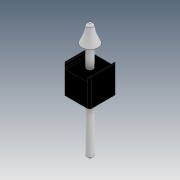
# Autodesk Inventor part: pins
Saved by Autodesk Inventor 2020 (Build 240168000, 168)
## iProperties
Created: 2020-09-27
Part Number: pins
Material: Generic
Document SubType Name: Modeling
Designer: DELL
Density: 1 g/cm^3
Appearance: Default
Author: DELL
Autodesk Inventor part; units mm, degrees
ref_plane "YZ Plane" through (0, 0, 0) normal (1, 0, 0) x (0, 1, 0)
ref_plane "XZ Plane" through (0, 0, 0) normal (0, 1, 0) x (-1, 0, 0)
sketch "Sketch5" plane through (0, 0, 0) normal (0, 1, 0) x (-1, 0, 0)
  line L0 (-1.225, -1.1) -> (1.225, -1.1)
  line L1 (1.225, -1.1) -> (1.225, 1.1)
  line L2 (1.225, 1.1) -> (-1.225, 1.1)
  line L3 (-1.225, 1.1) -> (-1.225, -1.1)
  line L4 (-1.225, -1.1) -> (1.225, 1.1) construction
  line L5 (1.225, -1.1) -> (-1.225, 1.1) construction
  line L6 (1.225, 1.1) -> (1.075, 1.27)
  line L7 (1.075, 1.27) -> (-1.075, 1.27)
  line L8 (-1.075, 1.27) -> (-1.225, 1.1)
  line L9 (0, 1.1) -> (0, -1.1) construction
  line L10 (1.225, 0) -> (-1.225, 0) construction
  line L11 (1.225, -1.1) -> (1.075, -1.27)
  line L12 (1.075, -1.27) -> (-1.075, -1.27)
  line L13 (-1.075, -1.27) -> (-1.225, -1.1)
  point P0 (0, 0)
  dimension "d33" = 2.2
  dimension "d34" = 2.45
  dimension "d36" = 0.15
  dimension "d37" = 2.54
  constraints: 28 end point, 6 midpoint, 2 horizontal, 2 parallel, 2 symmetric about line, 1 perpendicular, 1 other
  measures "d33" distance of L0.end L1.end
  measures "d34" distance between parallel lines of L3 L1
  measures "d36" horizontal distance of L1.end L6.end
  measures "d37" distance between parallel lines of L12 L7
extrude "Extrusion4" add sketch "Sketch5" along normal blind 2.54
sketch "Sketch6" plane through (-1.075, 0, 1.27) normal (0, 0, 1) x (1, 0, 0)
  line L0 (0, 2.54) -> (2.15, 2.54) projected
  line L1 (2.15, 2.14) -> (0, 2.14)
  line L2 (0, 2.14) -> (0, 2.54)
  line L3 (0, 2.54) -> (2.15, 2.54)
  line L4 (2.15, 2.54) -> (2.15, 2.14)
  line L5 (2.15, 2.14) -> (0, 2.54) construction
  line L6 (0, 2.14) -> (2.15, 2.54) construction
  line L7 (1.075, 0) -> (1.075, 2.54) construction
  point P0 (1.075, 2.34)
  dimension "d40" = 2.15
  dimension "d41" = 0.4
  constraints: 14 end point, 3 midpoint, 2 parallel, 2 perpendicular, 1 horizontal, 1 point on line, 1 other
  measures "d40" distance of L1.start L1.end
  measures "d41" distance of L3.end L1.start
extrude "Extrusion5" cut sketch "Sketch6" against normal through all
chamfer "Chamfer3" distance 0.1 angle 45 2 edges at (-1.075, 2.14, 0) (1.075, 2.14, 0)
chamfer "Chamfer4" distance 0.03 angle 45 2 edges at (1.075, 2.54, 0) (-1.075, 2.54, 0)
sketch "Sketch7" plane through (-0.975, 2.14, 1.27) normal (0, 1, 0) x (1, 0, 0)
  circle A0 centre (0.975, 1.27) radius 0.3
  dimension "d50" = 0.6
  constraints: 1 centre point, 1 coincident
  measures "d50" diameter of A0
extrude "Extrusion6" add sketch "Sketch7" along normal blind 3.6 and the other way blind 7.2
chamfer "Chamfer5" distance 0.2 angle 45 2 edges at (-0.3, 5.74, 0) (-0.3, -5.06, 0)
ref_plane "Work Plane1" through (0, 2.14, 0) normal (0, 0, -1) x (0, 1, 0)
sketch "Sketch8" plane through (0, 2.14, 0) normal (0, 0, -1) x (0, 1, 0)
  line L0 (0, -0.3) -> (3.4, -0.3) projected
  line L1 (1.975, -0.75) -> (1.975, 0)
  line L2 (3.4, 0) -> (3.4, -0.3)
  line L3 (0, 0.3) -> (0, -0.3) projected
  line L4 (3.4, -0.3) -> (3.4, 0.3) projected
  line L5 (3.6, 0.1) -> (3.6, -0.1) construction
  line L6 (3.6, 0) -> (0, 0) construction
  line L7 (-9.36, 0) -> (5.76, 0) construction
  line L8 (0.4, -1.225) -> (0.4, -1.105) construction
  line L9 (3.4, -0.3) -> (3.4, 0.3) projected
  line L10 (3.4, 0) -> (1.975, 0)
  line L11 (3.4, -0.3) -> (2.9466, -0.3) construction
  line L12 (2.9466, -0.3) -> (2.3806, -0.5247) construction
  line L13 (2.3806, -0.5247) -> (1.975, -0.75) construction
  spline S0 degree 3 poles (3.4, -0.3) (2.9466, -0.3) (2.3806, -0.5247) (1.975, -0.75) knots 1 1 1 1 2 2 2 2
  point P0 (-2.14, 0)
  point P1 (1.975, -0.3)
  dimension "d59" = 1.575
  dimension "d61" = 0.75
  constraints: 8 end point, 3 midpoint, 2 point on line, 1 collinear, 1 horizontal, 1 parallel, 1 perpendicular, 3 other
  measures "d59" distance between parallel lines of L1 L8
  measures "d61" distance of L1.start L1.end
revolve "Revolution1" add sketch "Sketch8" angle 360 about axis through (0, 2.14, 0) along (0, 1, 0) contours L0 S0 L1
body "Solid2"
